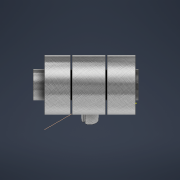
# Autodesk Inventor part: McCrea_rameno_Walle
Saved by Autodesk Inventor 2022 (Build 260153000, 153)
## iProperties
Created: 2022-01-25
Part Number: McCrea_rameno_Walle
Material: Generic
Document SubType Name: Modeling
Designer: Lukas
Density: 1 g/cm^3
Appearance: Honed
Author: Lukas
Autodesk Inventor part; units mm, degrees
ref_plane "YZ Plane" through (0, 0, 0) normal (1, 0, 0) x (0, 1, 0)
ref_plane "XZ Plane" through (0, 0, 0) normal (0, 1, 0) x (-1, 0, 0)
ref_plane "XY Plane" through (0, 0, 0) normal (0, 0, 1) x (1, 0, 0)
sketch "Sketch1" plane through (0, 0, 0) normal (0, 1, 0) x (-1, 0, 0)
  circle A0 centre (0, 0) radius 1.5
  line L0 (-0.25, 1.479) -> (-0.25, -1.479)
  line L1 (0.25, 1.479) -> (0.25, -1.479)
  line L2 (0, -7.0882) -> (0, 2.9314) projected
  point P0 (-1.4457, -0.4)
  point P1 (1.4457, -0.4)
  point P2 (1.4967, 0.1)
  point P3 (-1.4967, 0.1)
  dimension "d0" = 3
  dimension "d21" = 0.5
  dimension "d23" = 0.25
  constraints: 4 end point, 4 point on circle, 1 centre point, 1 coincident
  measures "d0" diameter of A0
  measures "d21" distance between parallel lines of L1 L0
  measures "d23" distance between parallel lines of L2 L1
extrude "Extrusion1" add sketch "Sketch1" along normal blind 4
extrude "Extrusion2" cut sketch "Sketch1" along normal blind 2.6 contours L1 A0 L2 | L2 A0 L0
sketch "Sketch2" plane through (0, 4, 0) normal (0, 1, 0) x (1, 0, 0)
  line L0 (0, 0) -> (-5.6569, -5.6569)
  line L1 (0, 0) -> (8, 0) construction
  line L2 (0, 0) -> (5.6569, 5.6569)
  line L3 (-5.6569, -5.6569) -> (-9.381, -1.9327)
  line L4 (-9.381, -1.9327) -> (1.9327, 9.381)
  line L5 (1.9327, 9.381) -> (5.6569, 5.6569)
  line L6 (-2.4034, -2.4034) -> (-6.1275, 1.3208)
  line L7 (-2.2144, -2.2144) -> (-5.9386, 1.5097)
  line L8 (-2.2144, -2.2144) -> (1.9327, 1.9327)
  line L9 (1.9327, 1.9327) -> (-1.7914, 5.6569)
  line L10 (1.9327, 1.9327) -> (2.1215, 2.1215)
  line L11 (2.1215, 2.1215) -> (-1.6026, 5.8457)
  dimension "d7" = 8
  dimension "d8" = 135
  dimension "d9" = 8
  dimension "d13" = 0.267
  constraints: 24 end point, 9 point on line, 6 perpendicular, 1 equal length, 1 horizontal
  measures "d7" distance of L0.start L0.end
  measures "d8" angle of L0 L1
  measures "d9" distance of L0.start L2.end
  measures "d13" distance of L10.start L10.end
extrude "Extrusion3" add sketch "Sketch1" against normal blind 3.5 contours A0 L1 | L0 A0
revolve "Revolution1" add sketch "Sketch2" angle 360 about axis through (0, 4, 0) along (0.7071, 0, -0.7071)
revolve "Revolution2" cut sketch "Sketch2" angle 360 about axis through (0, 4, 0) along (-0.7071, 0, 0.7071) contours L0 L6 L4 L7
revolve "Revolution3" cut sketch "Sketch2" angle 360 about axis through (0, 4, 0) along (0.7071, 0, -0.7071) contours L9 L4 L11 L2
sketch "Sketch3" plane through (-5.6569, 4, 5.6569) normal (-0.7071, 0, 0.7071) x (0.7071, 0, 0.7071)
  circle A0 centre (0, 0) radius 2.75
  point P0 (0, -4)
  dimension "d16" = 5.5
  constraints: 1 centre point
  measures "d16" diameter of A0
extrude "Extrusion4" add sketch "Sketch3" along normal blind 2 and the other way blind 16.5
sketch "Sketch5" plane through (0, 0, 0) normal (1, 0, 0) x (0, 1, 0)
  point P0 (0, 0)
sketch "Sketch6" plane through (5.6569, 4, -5.6569) normal (0.7071, 0, -0.7071) x (-0.7071, 0, -0.7071)
  point P0 (0, -4)
body "Solid1"
